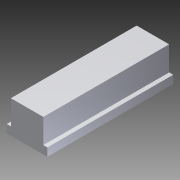
# Autodesk Inventor part: 8 ball plastic slider
Saved by Autodesk Inventor 2012 (Build 160160000, 160)
## iProperties
Created: 2013-10-15
Part Number: 8 ball plastic slider
Material: Default
Document SubType Name: Modeling
Designer: Bryce
Density: 1 g/cm^3
Author: Bryce
Autodesk Inventor part; units mm, degrees
ref_plane "YZ Plane" through (0, 0, 0) normal (1, 0, 0) x (0, 1, 0)
ref_plane "XZ Plane" through (0, 0, 0) normal (0, 1, 0) x (-1, 0, 0)
ref_plane "XY Plane" through (0, 0, 0) normal (0, 0, 1) x (1, 0, 0)
sketch "Sketch1" plane through (0, 0, 0) normal (0, 0, 1) x (1, 0, 0)
  line L0 (0, 0) -> (31.75, 0)
  line L1 (31.75, 0) -> (31.75, 6.35)
  line L2 (31.75, 25.4) -> (28.575, 25.4) construction
  line L3 (0, 25.4) -> (0, 6.35) construction
  line L4 (0, 6.35) -> (3.175, 6.35)
  line L5 (3.175, 6.35) -> (3.175, 25.4)
  line L6 (28.575, 25.4) -> (28.575, 6.35)
  line L7 (28.575, 6.35) -> (31.75, 6.35)
  line L8 (0, 6.35) -> (0, 0)
  line L9 (3.175, 25.4) -> (0, 25.4) construction
  line L10 (28.575, 25.4) -> (3.175, 25.4)
  line L11 (31.75, 6.35) -> (31.75, 25.4) construction
  dimension "d0" = 31.75
  dimension "d1" = 25.4
  dimension "d2" = 6.35
  dimension "d3" = 3.175
  constraints: 24 end point, 8 parallel, 6 perpendicular, 1 collinear, 1 horizontal, 1 horizontal alignment
  measures "d0" distance of L0.start L0.end
  measures "d1" distance of L3.start L0.start
  measures "d2" distance between parallel lines of L0 L4
  measures "d3" distance between parallel lines of L3 L5
extrude "Extrusion1" add sketch "Sketch1" along normal blind 98.425
body "Solid1"
